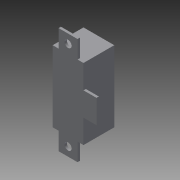
# Autodesk Inventor part: gp2
Saved by Autodesk Inventor 2015 (Build 190159000, 159)
## iProperties
Created: 2015-10-17
Part Number: gp2
Material: Générique
Document SubType Name: Modeling
Designer: astralien3000
Density: 1 g/cm^3
Appearance: Par défaut
Author: astralien3000
Autodesk Inventor part; units mm, degrees
ref_plane "YZ Plane" through (0, 0, 0) normal (1, 0, 0) x (0, 1, 0)
ref_plane "XZ Plane" through (0, 0, 0) normal (0, 1, 0) x (-1, 0, 0)
ref_plane "XY Plane" through (0, 0, 0) normal (0, 0, 1) x (1, 0, 0)
sketch "Esquisse1" plane through (0, 0, 0) normal (0, 1, 0) x (-1, 0, 0)
  line L0 (6.5, 15) -> (-6.5, 15)
  line L1 (-6.5, 15) -> (-6.5, -15)
  line L2 (-6.5, -15) -> (6.5, -15)
  line L3 (6.5, -15) -> (6.5, 15)
  line L4 (4, 15) -> (-4, 15)
  line L5 (-4, 15) -> (-4, 22.5)
  line L6 (-4, 22.5) -> (4, 22.5)
  line L7 (4, 22.5) -> (4, 15)
  line L8 (4, -15) -> (-4, -15)
  line L9 (-4, -15) -> (-4, -22.5)
  line L10 (-4, -22.5) -> (4, -22.5)
  line L11 (4, -22.5) -> (4, -15)
  line L12 (-6.5, -5) -> (-12, -5)
  line L13 (-12, -5) -> (-12, 5)
  line L14 (-12, 5) -> (-6.5, 5)
  line L15 (-6.5, 5) -> (-6.5, -5)
  point P0 (0, 0)
  dimension "d0" = 30
  dimension "d1" = 15
  dimension "d2" = 13
  dimension "d3" = 6.5
  dimension "d4" = 45
  dimension "d5" = 22.5
  dimension "d6" = 8
  dimension "d7" = 4
  dimension "d8" = 5.5
  dimension "d9" = 10
  dimension "d10" = 5
  constraints: 32 end point, 8 parallel, 5 point on line, 4 horizontal, 4 perpendicular
  measures "d0" distance of L2.end L0.start
  measures "d1" distance from line of L2 point (0, 0)
  measures "d2" distance of L0.start L0.end
  measures "d3" distance from line of point (0, 0) L3
  measures "d4" distance between parallel lines of L10 L6
  measures "d5" distance from line of point (0, 0) L10
  measures "d6" distance between parallel lines of L9 L11
  measures "d7" distance from line of point (0, 0) L11
  measures "d8" distance between parallel lines of L1 L13
  measures "d9" distance of L12.end L13.end
  measures "d10" distance from line of point (0, 0) L12
extrude "Extrusion1" add sketch "Esquisse1" along normal blind 1
sketch "Esquisse2" plane through (0, 1, 0) normal (0, 1, 0) x (1, 0, 0)
  line L0 (-6.5, -15) -> (6.5, -15)
  line L1 (6.5, -15) -> (6.5, 15)
  line L2 (6.5, 15) -> (-6.5, 15)
  line L3 (-6.5, 15) -> (-6.5, -15)
  point P0 (0, 0)
  constraints: 8 end point, 2 coincident, 2 parallel, 1 horizontal, 1 perpendicular
extrude "Extrusion2" add sketch "Esquisse2" along normal blind 12
sketch "Esquisse3" plane through (0, 0, 0) normal (0, -1, 0) x (1, 0, 0)
  line L0 (-4, 22.5) -> (4, 22.5) construction
  line L1 (4, 22.5) -> (4, 15) construction
  line L2 (4, 15) -> (-4, 15) construction
  line L3 (-4, 15) -> (-4, 22.5) construction
  line L4 (-4, -15) -> (4, -15) construction
  line L5 (4, -15) -> (4, -22.5) construction
  line L6 (4, -22.5) -> (-4, -22.5) construction
  line L7 (-4, -22.5) -> (-4, -15) construction
  line L8 (-4, 15) -> (4, 22.5) construction
  line L9 (4, 15) -> (-4, 22.5) construction
  line L10 (-4, -22.5) -> (4, -15) construction
  line L11 (-4, -15) -> (4, -22.5) construction
  circle A0 centre (0, -18.75) radius 1.5
  circle A1 centre (0, 18.75) radius 1.5
  point P0 (0, 0)
  dimension "d15" = 3
  dimension "d16" = 3
  constraints: 24 end point, 4 coincident, 4 parallel, 2 centre point, 2 horizontal, 2 midpoint, 2 perpendicular
  measures "d15" diameter of A1
  measures "d16" diameter of A0
extrude "Extrusion3" cut sketch "Esquisse3" against normal through all
equation "\"d1\" = 0.5 * d0"
equation "\"d3\" = 0.5 * d2"
equation "\"d5\" = 0.5 * d4"
equation "\"d7\" = 0.5 * d6"
equation "\"d10\" = 0.5 * d9"
equation "\"d16\" = d15"
